Autodesk Inventor part; units mm, degrees
(part 2 of 2)
  arc A88 (-113.7226, -29.3484) -> (-114.7619, -31.1484) centre (-113.7226, -30.5484) ccw
  line L237 (-113.7226, -29.3484) -> (-86.2786, -29.3484)
  line L238 (-85.2394, -31.1484) -> (-98.9614, -54.9156)
  line L239 (-101.0398, -54.9156) -> (-114.7619, -31.1484)
  circle A89 centre (-115.1083, -29.7484) radius 0.4 construction
  line L240 (-114.7619, -29.9484) -> (-115.4547, -29.5484) construction
  circle A90 centre (-116.6671, -28.8484) radius 3 construction
  line L241 (-100.0006, -28.8484) -> (-100.0006, -28.3484) construction
  line L242 (-114.7619, -29.9484) -> (-114.069, -30.3484) construction
  constraints: 1 horizontal, 28 other
extrude "Pixel Holes" cut sketch "Pixel Hole Sketch" against normal through all contours L13 A12 L14 A13 L12 A11 | L28 A17 L29 A18 L27 A16 | L43 A22 L44 A23 L42 A21 | L58 A27 L59 A28 L57 A26 | L73 A32 L74 A33 L72 A31 | L88 A37 L89 A38 L87 A36 | L103 A42 L104 A43 L102 A41 | L118 A47 L119 A48 L117 A46 | L133 A52 L134 A53 L132 A51 | L148 A57 L149 A58 L147 A56 | L163 A62 L164 A63 L162 A61 | L178 A67 L179 A68 L177 A66 | L193 A72 L194 A73 L192 A71 | L208 A77 L209 A78 L207 A76 | L223 A82 L224 A83 L222 A81 | L238 A87 L239 A88 L237 A86
equation "\"d24\" = Bolt_HeadDiameter"
equation "\"Base_SideWidth\" = 4 * Pixel_Stride"
body "Solid1"
